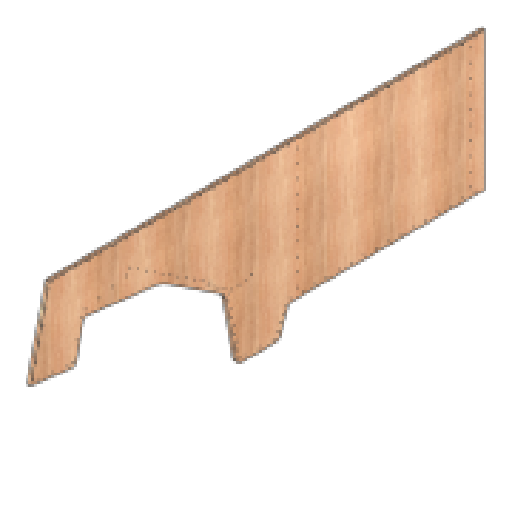
# Autodesk Inventor part: CUT PART A-01
Saved by Autodesk Inventor 2023.2 (Build 272271000, 271)
## iProperties
Created: 2022-11-02
Part Number: CUT PART A-01
Material: Wood (Birch)
Document SubType Name: Modeling
Designer: GUT
Density: 0.55 g/cm^3
Appearance: Birch - Natural Polished
Mass: 4432.57 g
Surface Area: 13971.5 cm^2
Volume: 8059.21 cm^3
Author: GUT
Autodesk Inventor part; units mm, degrees
ref_plane "YZ Plane" through (0, 0, 0) normal (1, 0, 0) x (0, 1, 0)
ref_plane "XZ Plane" through (0, 0, 0) normal (0, 1, 0) x (-1, 0, 0)
ref_plane "XY Plane" through (0, 0, 0) normal (0, 0, 1) x (1, 0, 0)
sketch "Sketch1" plane through (0, 0, 0) normal (1, 0, 0) x (0, 1, 0)
  line L0 (609.6339, -895.1116) -> (609.6339, 705.0745)
  line L1 (101.6046, -895.1116) -> (609.6339, -895.1116)
  line L2 (101.6046, -191.1252) -> (101.6046, -895.1116)
  line L3 (12.7452, -144.2404) -> (89.1216, -172.8816)
  line L4 (0, -1.0766) -> (0, -127.1818)
  line L5 (609.6339, 705.0745) -> (311.1839, 771.1144)
  line L6 (311.1839, 771.1144) -> (292.2034, 619.2706)
  line L7 (303.0756, 603.8577) -> (421.3918, 577.677)
  arc A0 (292.2471, 619.62) -> (303.1676, 603.8374) centre (306.105, 617.5393) ccw
  line L8 (432.2642, 562.2641) -> (401.9995, 320.1465)
  line L9 (12.7343, 15.3075) -> (229.8814, 56.0932)
  line L10 (382.5827, 267.2032) -> (256.3621, 73.9914)
  arc A1 (432.2642, 562.2641) -> (421.3918, 577.677) centre (418.3657, 564.0012) ccw
  arc A2 (382.5827, 267.2032) -> (401.9995, 320.1465) centre (277.7698, 335.6752) ccw
  arc A3 (229.8814, 56.0932) -> (256.3621, 73.9914) centre (222.4584, 95.6141) ccw
  arc A4 (12.7343, 15.3075) -> (0, -1.0766) centre (16.907, -1.0766) ccw
  arc A5 (0, -127.1818) -> (12.7452, -144.2404) centre (17.7886, -127.1818) ccw
  arc A6 (101.6046, -191.1252) -> (89.1216, -172.8816) centre (82.366, -190.8966) ccw
  point P0 (0, 0)
  constraints: 22 end point, 14 point on circle, 7 centre point, 6 tangent, 2 point on line
extrude "Extrusion1" add sketch "Sketch1" along normal blind 12
sketch "Sketch3" plane through (12, 0, 0) normal (1, 0, 0) x (0, 0, -1)
  line L0 (-771.1144, 311.1839) -> (-619.62, 292.2471) projected
  arc A0 (-619.62, 292.2471) -> (-603.8374, 303.1676) centre (-617.5393, 306.105) ccw projected
  line L1 (-603.8374, 303.1676) -> (-577.677, 421.3918) projected
  arc A1 (-562.2641, 432.2642) -> (-577.677, 421.3918) centre (-564.0012, 418.3657) ccw projected
  line L2 (-562.2641, 432.2642) -> (-320.1465, 401.9995) projected
  arc A2 (-267.2032, 382.5827) -> (-320.1465, 401.9995) centre (-335.6752, 277.7698) ccw projected
  line L3 (-267.2032, 382.5827) -> (-73.9914, 256.3621) projected
  arc A3 (-56.0932, 229.8814) -> (-73.9914, 256.3621) centre (-95.6141, 222.4584) ccw projected
  line L4 (-56.0932, 229.8814) -> (-15.3075, 12.7343) projected
  arc A4 (-15.3075, 12.7343) -> (1.0766, 0) centre (1.0766, 16.907) ccw projected
  line L5 (1.0766, 0) -> (127.1818, 0) projected
  arc A5 (127.1818, 0) -> (144.2404, 12.7452) centre (127.1818, 17.7886) ccw projected
  line L6 (144.2404, 12.7452) -> (172.8816, 89.1216) projected
  arc A6 (191.1252, 101.6046) -> (172.8816, 89.1216) centre (190.8966, 82.366) ccw projected
  line L7 (191.1252, 101.6046) -> (895.1116, 101.6046) projected
  line L8 (895.1116, 101.6046) -> (895.1116, 609.6339) projected
  line L9 (895.1116, 609.6339) -> (-705.0745, 609.6339) projected
  line L10 (-705.0745, 609.6339) -> (-771.1144, 311.1839) projected
  line L11 (52.0621, 255.3612) -> (-39.3397, 238.1937) projected
  line L12 (-39.3397, 238.1937) -> (-41.5548, 249.9875) projected
  line L13 (49.8469, 267.155) -> (-41.5548, 249.9875) projected
  line L14 (52.0621, 255.3612) -> (49.8469, 267.155) projected
  line L15 (5.8561, 20) -> (130.8561, 20) projected
  line L16 (130.8561, 20) -> (130.8561, 8) projected
  line L17 (5.8561, 8) -> (130.8561, 8) projected
  line L18 (5.8561, 20) -> (5.8561, 8) projected
  line L19 (-42.4778, 254.9015) -> (3.8561, 8.2152) projected
  line L20 (3.8561, 8.2152) -> (-7.9377, 6) projected
  line L21 (-54.2716, 252.6864) -> (-7.9377, 6) projected
  line L22 (-42.4778, 254.9015) -> (-54.2716, 252.6864) projected
  line L23 (128.8804, 23.0493) -> (161.535, 110.1279) projected
  line L24 (161.535, 110.1279) -> (172.7709, 105.9144) projected
  line L25 (140.1164, 18.8358) -> (172.7709, 105.9144) projected
  line L26 (128.8804, 23.0493) -> (140.1164, 18.8358) projected
  line L27 (213.1116, 588.6046) -> (213.1116, 124.6046) projected
  line L28 (213.1116, 124.6046) -> (201.1116, 124.6046) projected
  line L29 (201.1116, 588.6046) -> (201.1116, 124.6046) projected
  line L30 (213.1116, 588.6046) -> (201.1116, 588.6046) projected
  line L31 (870.1116, 107.6046) -> (171.1116, 107.6046) projected
  line L32 (171.1116, 107.6046) -> (171.1116, 119.6046) projected
  line L33 (870.1116, 119.6046) -> (171.1116, 119.6046) projected
  line L34 (870.1116, 107.6046) -> (870.1116, 119.6046) projected
  line L35 (870.1116, 597.6339) -> (-704.8884, 597.6339) projected
  line L36 (-704.8884, 597.6339) -> (-704.8884, 609.6339) projected
  line L37 (870.1116, 609.6339) -> (-704.8884, 609.6339) projected
  line L38 (870.1116, 597.6339) -> (870.1116, 609.6339) projected
  line L39 (-580.781, 457.7267) -> (-409.3081, 492.6843) projected
  line L40 (-409.3081, 492.6843) -> (-406.911, 480.9261) projected
  line L41 (-578.3839, 445.9685) -> (-406.911, 480.9261) projected
  line L42 (-580.781, 457.7267) -> (-578.3839, 445.9685) projected
  line L43 (-754.9801, 327.3072) -> (-623.0072, 310.8105) projected
  line L44 (-623.0072, 310.8105) -> (-624.4956, 298.9032) projected
  line L45 (-756.4685, 315.3998) -> (-624.4956, 298.9032) projected
  line L46 (-754.9801, 327.3072) -> (-756.4685, 315.3998) projected
  line L47 (-623.1563, 299.1747) -> (-590.1005, 448.5611) projected
  line L48 (-590.1005, 448.5611) -> (-578.3839, 445.9685) projected
  line L49 (-611.4397, 296.5821) -> (-578.3839, 445.9685) projected
  line L50 (-623.1563, 299.1747) -> (-611.4397, 296.5821) projected
  line L51 (-696.5215, 592.7442) -> (-758.0958, 314.4752) projected
  line L52 (-758.0958, 314.4752) -> (-769.8124, 317.0678) projected
  line L53 (-708.2381, 595.3368) -> (-769.8124, 317.0678) projected
  line L54 (-696.5215, 592.7442) -> (-708.2381, 595.3368) projected
  line L55 (-409.9271, 513.6948) -> (-100.1674, 311.3364) projected
  line L56 (-100.1674, 311.3364) -> (-106.7304, 301.2901) projected
  line L57 (-416.4901, 503.6485) -> (-106.7304, 301.2901) projected
  line L58 (-409.9271, 513.6948) -> (-416.4901, 503.6485) projected
  line L59 (-125.5671, 313.5957) -> (-47.7086, 262.7326) projected
  line L60 (-47.7086, 262.7326) -> (-54.2716, 252.6864) projected
  line L61 (-132.1301, 303.5494) -> (-54.2716, 252.6864) projected
  line L62 (-125.5671, 313.5957) -> (-132.1301, 303.5494) projected
  line L63 (850.1116, 588.6046) -> (850.1116, 124.6046) projected
  line L64 (850.1116, 124.6046) -> (838.1116, 124.6046) projected
  line L65 (838.1116, 588.6046) -> (838.1116, 124.6046) projected
  line L66 (850.1116, 588.6046) -> (838.1116, 588.6046) projected
  line L67 (213.1116, 588.6046) -> (213.1116, 124.6046) projected
  line L68 (213.1116, 124.6046) -> (201.1116, 124.6046) projected
  line L69 (201.1116, 588.6046) -> (201.1116, 124.6046) projected
  line L70 (213.1116, 588.6046) -> (201.1116, 588.6046) projected
  point P0 (860.1116, 113.6046)
  point P1 (844.1116, 134.6046)
  point P2 (860.1116, 603.6339)
  point P3 (207.1116, 134.6046)
  point P4 (163.6417, 98.6579)
  point P5 (120.8561, 14)
  point P6 (41.1263, 259.4122)
  point P7 (-3.8868, 16.9357)
  point P8 (-59.362, 263.1787)
  point P9 (-111.8208, 311.7824)
  point P10 (-417.908, 484.8076)
  point P11 (-586.4027, 437.501)
  point P12 (-633.6742, 306.0972)
  point P13 (-761.7936, 325.5353)
  point P14 (844.1116, 183.938)
  point P15 (844.1116, 233.2713)
  point P16 (844.1116, 282.6046)
  point P17 (844.1116, 331.938)
  point P18 (844.1116, 381.2713)
  point P19 (814.8449, 113.6046)
  point P20 (769.5783, 113.6046)
  point P21 (724.3116, 113.6046)
  point P22 (679.0449, 113.6046)
  point P23 (633.7783, 113.6046)
  point P24 (588.5116, 113.6046)
  point P25 (543.2449, 113.6046)
  point P26 (497.9783, 113.6046)
  point P27 (844.1116, 183.938)
  point P28 (207.1116, 183.938)
  point P29 (844.1116, 233.2713)
  point P30 (207.1116, 233.2713)
  point P31 (844.1116, 282.6046)
  point P32 (207.1116, 282.6046)
  point P33 (844.1116, 331.938)
  point P34 (207.1116, 331.938)
  point P35 (844.1116, 381.2713)
  point P36 (207.1116, 381.2713)
  point P37 (814.3763, 603.6339)
  point P38 (768.641, 603.6339)
  point P39 (722.9057, 603.6339)
  point P40 (677.1704, 603.6339)
  point P41 (631.4351, 603.6339)
  point P42 (585.6998, 603.6339)
  point P43 (539.9645, 603.6339)
  point P44 (494.2292, 603.6339)
  point P45 (448.494, 603.6339)
  point P46 (402.7587, 603.6339)
  point P47 (357.0234, 603.6339)
  point P48 (311.2881, 603.6339)
  point P49 (265.5528, 603.6339)
  point P50 (219.8175, 603.6339)
  point P51 (174.0822, 603.6339)
  point P52 (128.3469, 603.6339)
  point P53 (82.6116, 603.6339)
  point P54 (36.8763, 603.6339)
  point P55 (-8.859, 603.6339)
  point P56 (155.0977, 75.8738)
  point P57 (17.2112, 254.9203)
  point P58 (-79.7336, 276.4869)
  point P59 (68.3561, 14)
  point P60 (-9.217, 45.3145)
  point P61 (-14.5473, 73.6932)
  point P62 (-19.8775, 102.072)
  point P63 (-141.1224, 330.9244)
  point P64 (-170.424, 350.0664)
  point P65 (-199.7256, 369.2084)
  point P66 (-229.0272, 388.3504)
  point P67 (-258.3288, 407.4925)
  point P68 (-287.6303, 426.6345)
  point P69 (-316.9319, 445.7765)
  point P70 (-468.5333, 474.4868)
  point P71 (-600.7701, 372.5716)
  point P72 (-689.7379, 313.1052)
  point P73 (-750.3429, 377.2836)
  point P74 (-738.8923, 429.0319)
  point P75 (-727.4416, 480.7801)
  point P76 (-25.2077, 130.4508)
  point P77 (-30.538, 158.8295)
  point P78 (-715.9909, 532.5284)
  point P79 (-54.5943, 603.6339)
  point P80 (-100.3296, 603.6339)
  point P81 (-146.0649, 603.6339)
  point P82 (-191.8002, 603.6339)
  point P83 (-237.5355, 603.6339)
  point P84 (-283.2708, 603.6339)
  point P85 (-519.1586, 464.166)
  point P86 (452.7116, 113.6046)
  point P87 (407.4449, 113.6046)
  point P88 (362.1783, 113.6046)
  point P89 (844.1116, 430.6046)
  point P90 (844.1116, 479.938)
  point P91 (-35.8682, 187.2083)
  point P92 (146.5537, 53.0898)
  point P93 (138.0097, 30.3058)
  point P94 (-346.2335, 464.9185)
  point P95 (844.1116, 430.6046)
  point P96 (207.1116, 430.6046)
  point P97 (844.1116, 479.938)
  point P98 (207.1116, 479.938)
  point P99 (-100.1051, 289.7952)
  point P100 (-120.4767, 303.1034)
  point P101 (-6.704, 250.4284)
  point P102 (-30.6191, 245.9366)
  point P103 (-704.5403, 584.2766)
  point P104 (15.8561, 14)
  point P105 (-329.006, 603.6339)
  point P106 (-374.7413, 603.6339)
  point P107 (-420.4766, 603.6339)
  point P108 (-466.2119, 603.6339)
  point P109 (-511.9472, 603.6339)
  point P110 (-557.6825, 603.6339)
  point P111 (-603.4178, 603.6339)
  point P112 (-649.1531, 603.6339)
  point P113 (-694.8884, 603.6339)
  point P114 (-569.784, 453.8452)
  point P115 (316.9116, 113.6046)
  point P116 (271.6449, 113.6046)
  point P117 (226.3783, 113.6046)
  point P118 (181.1116, 113.6046)
  point P119 (844.1116, 529.2713)
  point P120 (844.1116, 578.6046)
  point P121 (-41.1985, 215.5871)
  point P122 (-46.5287, 243.9658)
  point P123 (-745.8015, 320.1131)
  point P124 (-615.1375, 307.6422)
  point P125 (-375.5351, 484.0605)
  point P126 (-404.8367, 503.2025)
  point P127 (844.1116, 529.2713)
  point P128 (207.1116, 529.2713)
  point P129 (844.1116, 578.6046)
  point P130 (207.1116, 578.6046)
  dimension "b" = 10
  dimension "a" = 6
  dimension "d156" = 6
  dimension "d157" = 10
  dimension "d158" = 6
  dimension "d159" = 10
  dimension "d160" = 6
  dimension "d161" = 10
  dimension "d162" = 6
  dimension "d163" = 10
  dimension "d164" = 6
  dimension "d165" = 10
  dimension "d166" = 6
  dimension "d167" = 10
  dimension "d168" = 6
  dimension "d169" = 10
  dimension "d170" = 6
  dimension "d171" = 10
  dimension "d172" = 10
  dimension "d173" = 6
  dimension "d174" = 6
  dimension "d175" = 10
  dimension "d176" = 6
  dimension "d177" = 10
  dimension "d178" = 6
  dimension "d179" = 10
  dimension "d180" = 10
  dimension "d181" = 6
  dimension "d184" = 49.3333
  dimension "d191" = 45.2667
  dimension "d198" = 49.3333
  dimension "d205" = 45.7353
  dimension "d212" = 24.3333
  dimension "d219" = 24.3333
  dimension "d226" = 24.3333
  dimension "d233" = 52.5
  dimension "d240" = 28.875
  dimension "d247" = 35
  dimension "d254" = 51.6667
  dimension "d261" = 66.5
  dimension "d268" = 56.5
  dimension "d275" = 53
  constraints: 3 horizontal, 2 vertical, 127 other
  measures "b" distance from line of L34 point (860.112, 113.605)
  measures "a" distance from line of L31 point (860.112, 113.605)
  measures "d156" distance from line of L65 point (844.112, 134.605)
  measures "d157" distance from line of L64 point (844.112, 134.605)
  measures "d158" distance from line of L35 point (860.112, 603.634)
  measures "d159" distance from line of L38 point (860.112, 603.634)
  measures "d160" distance from line of L29 point (207.112, 134.605)
  measures "d161" distance from line of L68 point (207.112, 134.605)
  measures "d162" distance from line of L23 point (163.642, 98.658)
  measures "d164" distance from line of L15 point (120.856, 14)
  measures "d165" distance from line of L16 point (120.856, 14)
  measures "d166" distance from line of L13 point (41.126, 259.412)
  measures "d167" distance from line of L14 point (41.126, 259.412)
  measures "d168" distance from line of L21 point (-3.887, 16.936)
  measures "d169" distance from line of L20 point (-3.887, 16.936)
  measures "d170" distance from line of L59 point (-59.362, 263.179)
  measures "d171" distance from line of L60 point (-59.362, 263.179)
  measures "d172" distance from line of L56 point (-111.821, 311.782)
  measures "d173" distance from line of L55 point (-111.821, 311.782)
  measures "d174" distance from line of L39 point (-417.908, 484.808)
  measures "d175" distance from line of L40 point (-417.908, 484.808)
  measures "d176" distance from line of L47 point (-586.403, 437.501)
  measures "d177" distance from line of point (-586.403, 437.501) L48
  measures "d178" distance from line of L43 point (-633.674, 306.097)
  measures "d179" distance from line of L44 point (-633.674, 306.097)
  measures "d180" distance from line of L52 point (-761.794, 325.535)
  measures "d181" distance from line of L53 point (-761.794, 325.535)
  measures "d184" distance of point (844.112, 134.605) point (844.112, 183.938)
  measures "d191" distance of point (860.112, 113.605) point (814.845, 113.605)
  measures "d198" distance of point (844.112, 134.605) point (844.112, 183.938)
  measures "d205" distance of point (860.112, 603.634) point (814.376, 603.634)
  measures "d212" distance of point (163.642, 98.658) point (155.098, 75.874)
  measures "d219" distance of point (41.126, 259.412) point (17.211, 254.92)
  measures "d226" distance of point (-59.362, 263.179) point (-79.734, 276.487)
  measures "d233" distance of point (120.856, 14) point (68.356, 14)
  measures "d240" distance of point (-3.887, 16.936) point (-9.217, 45.314)
  measures "d247" distance of point (-111.821, 311.782) point (-141.122, 330.924)
  measures "d254" distance of point (-417.908, 484.808) point (-468.533, 474.487)
  measures "d261" distance of point (-586.403, 437.501) point (-600.77, 372.572)
  measures "d268" distance of point (-633.674, 306.097) point (-689.738, 313.105)
  measures "d275" distance of point (-761.794, 325.535) point (-750.343, 377.284)
hole "Hole4" at (12, 113.6046, -860.1116) at (12, 134.6046, -844.1116) at (12, 603.6339, -860.1116) at (12, 134.6046, -207.1116) at (12, 98.6579, -163.6417) at (12, 14, -120.8561) at (12, 259.4122, -41.1263) at (12, 16.9357, 3.8868) at (12, 263.1787, 59.362) at (12, 311.7824, 111.8208) at (12, 484.8076, 417.908) at (12, 437.501, 586.4027) at (12, 306.0972, 633.6742) at (12, 325.5353, 761.7936) at (12, 183.938, -844.1116) at (12, 233.2713, -844.1116) at (12, 282.6046, -844.1116) at (12, 331.938, -844.1116) at (12, 381.2713, -844.1116) at (12, 113.6046, -814.8449) at (12, 113.6046, -769.5783) at (12, 113.6046, -724.3116) at (12, 113.6046, -679.0449) at (12, 113.6046, -633.7783) at (12, 113.6046, -588.5116) at (12, 113.6046, -543.2449) at (12, 113.6046, -497.9783) at (12, 183.938, -207.1116) at (12, 233.2713, -207.1116) at (12, 282.6046, -207.1116) at (12, 331.938, -207.1116) at (12, 381.2713, -207.1116) at (12, 603.6339, -814.3763) at (12, 603.6339, -768.641) at (12, 603.6339, -722.9057) at (12, 603.6339, -677.1704) at (12, 603.6339, -631.4351) at (12, 603.6339, -585.6998) at (12, 603.6339, -539.9645) at (12, 603.6339, -494.2292) at (12, 603.6339, -448.494) at (12, 603.6339, -402.7587) at (12, 603.6339, -357.0234) at (12, 603.6339, -311.2881) at (12, 603.6339, -265.5528) at (12, 603.6339, -219.8175) at (12, 603.6339, -174.0822) at (12, 603.6339, -128.3469) at (12, 603.6339, -82.6116) at (12, 603.6339, -36.8763) direction (-1, 0, 0) diameter 3.5 end through all and at (12, 603.6339, 8.859) (12, 75.8738, -155.0977) (12, 254.9203, -17.2112) (12, 276.4869, 79.7336) (12, 14, -68.3561) (12, 45.3145, 9.217) (12, 73.6932, 14.5473) (12, 102.072, 19.8775) (12, 330.9244, 141.1224) (12, 350.0664, 170.424) (12, 369.2084, 199.7256) (12, 388.3504, 229.0272) (12, 407.4925, 258.3288) (12, 426.6345, 287.6303) (12, 445.7765, 316.9319) (12, 474.4868, 468.5333) (12, 372.5716, 600.7701) (12, 313.1052, 689.7379) (12, 377.2836, 750.3429) (12, 429.0319, 738.8923) (12, 480.7801, 727.4416) (12, 130.4508, 25.2077) (12, 158.8295, 30.538) (12, 532.5284, 715.9909) (12, 603.6339, 54.5943) (12, 603.6339, 100.3296) (12, 603.6339, 146.0649) (12, 603.6339, 191.8002) (12, 603.6339, 237.5355) (12, 603.6339, 283.2708) (12, 464.166, 519.1586) (12, 113.6046, -452.7116) (12, 113.6046, -407.4449) (12, 113.6046, -362.1783) (12, 430.6046, -844.1116) (12, 479.938, -844.1116) (12, 187.2083, 35.8682) (12, 53.0898, -146.5537) (12, 30.3058, -138.0097) (12, 464.9185, 346.2335) (12, 430.6046, -207.1116) (12, 479.938, -207.1116) (12, 289.7952, 100.1051) (12, 303.1034, 120.4767) (12, 250.4284, 6.704) (12, 245.9366, 30.6191) (12, 584.2766, 704.5403) (12, 14, -15.8561) (12, 603.6339, 329.006) (12, 603.6339, 374.7413) (12, 603.6339, 420.4766) (12, 603.6339, 466.2119) (12, 603.6339, 511.9472) (12, 603.6339, 557.6825) (12, 603.6339, 603.4178) (12, 603.6339, 649.1531) (12, 603.6339, 694.8884) (12, 453.8452, 569.784) (12, 113.6046, -316.9116) (12, 113.6046, -271.6449) (12, 113.6046, -226.3783) (12, 113.6046, -181.1116) (12, 529.2713, -844.1116) (12, 578.6046, -844.1116) (12, 215.5871, 41.1985) (12, 243.9658, 46.5287) (12, 320.1131, 745.8015) (12, 307.6422, 615.1375) (12, 484.0605, 375.5351) (12, 503.2025, 404.8367) (12, 529.2713, -207.1116) (12, 578.6046, -207.1116)
equation "\"d156\" = a"
equation "\"d157\" = b"
equation "\"d158\" = a"
equation "\"d159\" = b"
equation "\"d160\" = a"
equation "\"d161\" = b"
equation "\"d162\" = a"
equation "\"d163\" = b"
equation "\"d164\" = a"
equation "\"d165\" = b"
equation "\"d166\" = a"
equation "\"d167\" = b"
equation "\"d168\" = a"
equation "\"d169\" = b"
equation "\"d171\" = b"
equation "\"d172\" = b"
equation "\"d173\" = a"
equation "\"d174\" = a"
equation "\"d175\" = b"
equation "\"d176\" = a"
equation "\"d177\" = b"
equation "\"d178\" = a"
equation "\"d179\" = b"
equation "\"d180\" = b"
equation "\"d181\" = a"
equation "\"wsp\" = 45"
body "Solid1"
